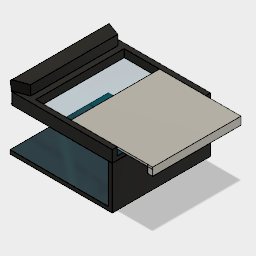
Hologram unit (Autodesk Fusion 360 design; units mm, degrees)
Autodesk Fusion 360 part; units mm, degrees
note: some values were not read from the file. Chosen so that the rebuilt part matches the saved one: that a step has no effect; the sign of a taper.
sketch "Sketch1" plane through (0, 0, 0) normal (0, 1, 0) x (1, 0, 0)
  line L0 (1.3, 0.4) -> (6.3, 0.4)
  line L1 (6.3, 0.4) -> (6.3, 5.4)
  line L2 (6.3, 5.4) -> (1.3, 5.4)
  line L3 (1.3, 5.4) -> (1.3, 0.4)
  dimension "d1" = 5
  dimension "d2" = 5
  measures "d1" distance of L0.start L0.end
  measures "d2" distance of L0.start L2.end
extrude "Extrude1" add sketch "Sketch1" along normal blind 2 draft -45 makes body 1
sketch "Sketch2" plane through (0, 0, 0) normal (0, -1, 0) x (1, 0, 0)
  line L0 (1.3, -0.4) -> (1.3, -5.4)
  line L1 (1.3, -5.4) -> (6.3, -5.4)
  line L2 (6.3, -5.4) -> (6.3, -0.4)
  line L3 (6.3, -0.4) -> (1.3, -0.4)
  line L4 (1.3, -0.4) -> (6.3, -0.4)
  line L5 (6.3, -0.4) -> (6.3, -5.4)
  line L6 (6.3, -5.4) -> (1.3, -5.4)
  line L7 (1.3, -5.4) -> (1.3, -0.4)
extrude "Extrude2" add sketch "Sketch2" along normal blind 0.2 bodies 1
extrude "Extrude3" add 1 faces at (6.3, -0.1333, -3.7333) along direction (1, 0, 0) blind 0.3 on bodies 1 bodies 1
extrude "Extrude4" add 1 faces at (6.4, 0, -2.0667) along direction (0, 1, 0) blind 2 on bodies 1 bodies 1
move_face "OffsetFaces1" offset -0.1 1 faces at (6.6, 1.2667, -3.7333) on bodies 1
sketch "Sketch1 (2)" plane through (0, -0.2, 0) normal (0, -1, 0) x (1, 0, 0) in component "Component"
  line L0 (1.3, -5.4) -> (6.5, -5.4)
  line L1 (6.5, -5.4) -> (6.5, -0.4)
  line L2 (6.5, -0.4) -> (1.3, -0.4)
  line L3 (1.3, -0.4) -> (1.3, -5.4)
  line L4 (1.3, -5.4) -> (6.5, -5.4)
  line L5 (6.5, -5.4) -> (6.5, -0.4)
  line L6 (6.5, -0.4) -> (1.3, -0.4)
  line L7 (1.3, -0.4) -> (1.3, -5.4)
extrude "Extrude1'" add sketch "Sketch1 (2)" along normal blind 0.3 separate body makes body 2 in component "Component"
move_face "OffsetFaces1'" offset 0.3 1 faces at (3.0333, -0.2, -2.0667) on bodies 2 in component "Component"
sketch "Sketch2 (2)" plane through (0, 0.1, 0) normal (0, 1, 0) x (-1, 0, 0) in component "Component"
  line L0 (-1.3, -5.4) -> (-1.3, -0.4)
  line L1 (-1.3, -0.4) -> (-6.5, -0.4)
  line L2 (-6.5, -0.4) -> (-6.5, -5.4)
  line L3 (-6.5, -5.4) -> (-1.3, -5.4)
  line L4 (-1.5531, -0.6531) -> (-6.2469, -0.6531)
  line L5 (-6.2469, -0.6531) -> (-6.2469, -5.1469)
  line L6 (-6.2469, -5.1469) -> (-1.5531, -5.1469)
  line L7 (-1.5531, -5.1469) -> (-1.5531, -0.6531)
  dimension "d17" = 0.2531
extrude "Extrude2'" cut sketch "Sketch2 (2)" against normal blind 0.4 contours L4 L5 L6 L7 bodies 2 in component "Component"
sketch "Sketch4" plane through (0, 2.2, 0) normal (0, 1, 0) x (-1, 0, 0)
  line L0 (-1.5531, -5.1469) -> (-1.5531, -0.6531)
  line L1 (-1.5531, -0.6531) -> (-6.2469, -0.6531)
  line L2 (-6.2469, -0.6531) -> (-6.2469, -5.1469)
  line L3 (-6.2469, -5.1469) -> (-1.5531, -5.1469)
  line L4 (-1.5531, -5.1469) -> (-2.3552, -5.1469)
  line L5 (-2.3552, -5.1469) -> (-2.3552, -0.6531)
  line L6 (-2.3552, -0.6531) -> (-1.5531, -0.6531)
  line L7 (-1.5531, -0.6531) -> (-1.5531, -5.1469)
extrude "Extrude3'" add sketch "Sketch4" along normal blind 0.4 contours L0 L1 L3 L4 L5 L6 L7 sketch seen with x (1, 0, 0) y (0, 1, 0) z (0, 0, 1) at (0, -2.5, 0) bodies 2 in component "Component"
sketch "Sketch5" plane through (0, 2.6, 0) normal (0, 1, 0) x (-1, 0, 0)
  line L0 (-6.2469, -0.6531) -> (-2.3552, -0.6531)
  line L1 (-2.3552, -0.6531) -> (-2.3552, -5.1469)
  line L2 (-2.3552, -5.1469) -> (-6.2469, -5.1469)
  line L3 (-6.2469, -5.1469) -> (-6.2469, -0.6531)
  line L4 (-1.3, -5.4) -> (-1.3, -0.4)
  line L5 (-1.3, -0.4) -> (-6.5, -0.4)
  line L6 (-6.5, -0.4) -> (-6.5, -5.4)
  line L7 (-6.5, -5.4) -> (-1.3, -5.4)
  line L8 (-6.2469, -5.1469) -> (-6.5, -5.1469)
  line L9 (-6.5, -5.1469) -> (-6.5, -0.6503)
  line L10 (-6.5, -0.6503) -> (-6.2469, -0.6503)
  line L11 (-6.2469, -0.6503) -> (-6.2469, -5.1469)
extrude "Extrude4'" cut sketch "Sketch5" against normal blind 0.4 contours L3 L6 L8 L9 L10 L11 sketch seen with x (1, 0, 0) y (0, 1, 0) z (0, 0, 1) at (0, -2.5, 0) bodies 2 in component "Component"
sketch "Sketch1 (3)" plane through (0, 2.6, 0) normal (0, 1, 0) x (-1, 0, 0) in component "Cover"
  line L0 (-6.5, -0.6503) -> (-6.2469, -0.6503)
  line L1 (-6.2469, -0.6503) -> (-6.2469, -0.6531)
  line L2 (-6.2469, -0.6531) -> (-2.3552, -0.6531)
  line L3 (-2.3552, -0.6531) -> (-2.3552, -5.1469)
  line L4 (-2.3552, -5.1469) -> (-6.5, -5.1469)
  line L5 (-6.5, -5.1469) -> (-6.5, -5.4)
  line L6 (-6.5, -5.4) -> (-1.3, -5.4)
  line L7 (-1.3, -5.4) -> (-1.3, -0.4)
  line L8 (-1.3, -0.4) -> (-6.5, -0.4)
  line L9 (-6.5, -0.4) -> (-6.5, -0.6503)
  line L10 (-2.3552, -5.1469) -> (-6.5, -5.1469)
  line L11 (-6.5, -5.1469) -> (-6.5, -0.6503)
  line L12 (-6.5, -0.6503) -> (-2.3552, -0.6503)
  line L13 (-2.3552, -0.6503) -> (-2.3552, -5.1469)
extrude "Extrude1''" add sketch "Sketch1 (3)" against normal blind 0.1 separate body contours L0 L1 L2 L3 L4 L10 L11 L12 L13 makes body 3 in component "Cover"
sketch "Sketch2 (3)" plane through (0, 2.5, 0) normal (0, -1, 0) x (1, 0, 0) in component "Cover"
  line L0 (6.2469, -0.6503) -> (6.2469, -0.6531)
  line L1 (6.2469, -0.6531) -> (2.3552, -0.6531)
  line L2 (2.3552, -0.6531) -> (2.3552, -5.1469)
  line L3 (2.3552, -5.1469) -> (6.5, -5.1469)
  line L4 (6.5, -5.1469) -> (6.5, -0.6503)
  line L5 (6.5, -0.6503) -> (6.2469, -0.6503)
  line L6 (6.2469, -0.6531) -> (6.5, -0.6531)
  line L7 (6.5, -0.6531) -> (6.5, -5.1469)
  line L8 (6.5, -5.1469) -> (6.2469, -5.1469)
  line L9 (6.2469, -5.1469) -> (6.2469, -0.6531)
extrude "Extrude2''" add sketch "Sketch2 (3)" along normal blind 0.3 contours L3 L4 L6 L7 L8 L9 bodies 3 in component "Cover"
move_body "Move1" bodies 3 to x (1, 0, 0) y (0, 1, 0) z (0, 0, 1) at (1.8, 0, 0) in component "Cover"
sketch "Sketch1 (4)" plane through (0, 2.6, 0) normal (0, 1, 0) x (-1, 0, 0) in component "Kinect"
  line L0 (-6.5, -0.6503) -> (-6.2469, -0.6503)
  line L1 (-6.2469, -0.6503) -> (-6.2469, -0.6531)
  line L2 (-6.2469, -0.6531) -> (-2.3552, -0.6531)
  line L3 (-2.3552, -0.6531) -> (-2.3552, -5.1469)
  line L4 (-2.3552, -5.1469) -> (-6.5, -5.1469)
  line L5 (-6.5, -5.1469) -> (-6.5, -5.4)
  line L6 (-6.5, -5.4) -> (-1.3, -5.4)
  line L7 (-1.3, -5.4) -> (-1.3, -0.4)
  line L8 (-1.3, -0.4) -> (-6.5, -0.4)
  line L9 (-6.5, -0.4) -> (-6.5, -0.6503)
  line L10 (-1.3, -5.4) -> (-2.069, -5.4)
  line L11 (-2.069, -5.4) -> (-2.069, -0.4)
  line L12 (-2.069, -0.4) -> (-1.3, -0.4)
  line L13 (-1.3, -0.4) -> (-1.3, -5.4)
extrude "Extrude1'''" add sketch "Sketch1 (4)" along normal blind 0.5 separate body contours L6 L7 L8 L10 L11 L12 L13 makes body 4 in component "Kinect"
form "Form1" [no effect] in component "Kinect"
draft "Draft2" angle -20 neutral plane through (1.3, 2.6, -5.4) pull (-1, 0, 0) 1 faces at (1.5563, 2.7667, -0.4) on bodies 4 in component "Kinect"
draft "Draft3" angle -20 neutral plane through (1.3, 2.6, -5.4) pull (-1, 0, 0) 1 faces at (1.8126, 2.7667, -5.4) on bodies 4 in component "Kinect"
draft "Draft4" angle 5 neutral plane through (0, 3.1, 0) pull (0, -1, 0) 1 faces at (1.3, 2.7667, -3.7333) on bodies 4 in component "Kinect"
fillet "Fillet1" radius 0.06 2 edges at (1.3, 3.1, -2.9) (1.3437, 2.6, -2.9) on bodies 4 in component "Kinect"
sketch "Sketch4 (2)" plane through (1.5593, 0.1364, 0) normal (-0.996195, -0.087156, 0) x (0, 0, 1) in component "Kinect"
  line L0 (-5.3858, 2.528) -> (-0.4142, 2.528)
  line L1 (-0.4142, 2.528) -> (-0.4021, 2.9094)
  line L2 (-0.4021, 2.9094) -> (-5.3979, 2.9094)
  line L3 (-5.3979, 2.9094) -> (-5.3858, 2.528)
  circle A0 centre (-4, 2.75) radius 0.15
  circle A1 centre (-2.85, 2.75) radius 0.15
  circle A2 centre (-2.3743, 2.7507) radius 0.15
  dimension "d41" = 0.3
  dimension "d42" = 0.3
  dimension "d43" = 0.3
  measures "d41" diameter of A0
  measures "d42" diameter of A1
  measures "d43" diameter of A2
extrude "Extrude3''" cut sketch "Sketch4 (2)" against normal blind 0.1 draft -30 contours A0 | A1 | A2 bodies 4 in component "Kinect"
fillet "Fillet1'" radius 0.1 1 edges at (1.3, -0.2, -0.4) on bodies 2 in component "Component"
fillet "Fillet2" radius 0.1 1 edges at (1.3, -0.2, -5.4) on bodies 2 in component "Component"
sketch "Sketch6" plane through (1.5593, 0.1364, 0) normal (-0.996195, -0.087156, 0) x (0, 0, 1)
  circle A0 centre (-4, 2.75) radius 0.15
  circle A1 centre (-2.85, 2.75) radius 0.15
  circle A2 centre (-2.3743, 2.7507) radius 0.15
  line L0 (-5.3858, 2.528) -> (-0.4142, 2.528)
  line L1 (-0.4142, 2.528) -> (-0.4021, 2.9094)
  line L2 (-0.4021, 2.9094) -> (-5.3979, 2.9094)
  line L3 (-5.3979, 2.9094) -> (-5.3858, 2.528)
  circle A3 centre (-4, 2.75) radius 0.15
  circle A4 centre (-4, 2.75) radius 0.15
  circle A5 centre (-2.85, 2.75) radius 0.15
  circle A6 centre (-2.3743, 2.7507) radius 0.15
  circle A7 centre (-3.55, 2.75) radius 0.0258
extrude "Extrude4''" cut sketch "Sketch6" against normal blind 0.01 contours A7 bodies 4 in component "Kinect"
sketch "Sketch1 (5)" plane through (0, 0, 0) normal (0, 1, 0) x (1, 0, 0) in component "Base"
  line L0 (6.5, 5.4) -> (1.3, 5.4)
  line L1 (1.3, 5.4) -> (1.3, 0.4)
  line L2 (1.3, 0.4) -> (6.5, 0.4)
  line L3 (6.5, 0.4) -> (6.5, 5.4)
  line L4 (6.5, 5.4) -> (6.3, 5.4)
  line L5 (6.3, 5.4) -> (6.3, 0.4)
  line L6 (6.3, 0.4) -> (6.5, 0.4)
  line L7 (6.5, 0.4) -> (6.5, 5.4)
  point P0 (6.5, 5.4)
  point P1 (1.3, 0.4)
  point P2 (6.3, 0.4)
extrude "Extrude1''''" add sketch "Sketch1 (5)" against normal blind 0.2 separate body contours L0 L1 L2 L5 makes body 5 in component "Base"
extrude "Extrude2'''" add 1 faces at (6.3, -0.0667, -3.7333) along direction (1, 0, 0) blind 0.2 on bodies 5 bodies 5 in component "Base"
sketch "Sketch2 (4)" plane through (0, 0, 0) normal (0, 1, 0) x (-1, 0, 0) in component "Base"
  line L0 (-1.3, -5.4) -> (-1.3, -0.4)
  line L1 (-1.3, -0.4) -> (-6.5, -0.4)
  line L2 (-6.5, -0.4) -> (-6.5, -5.4)
  line L3 (-6.5, -5.4) -> (-1.3, -5.4)
  line L4 (-6.5, -0.4) -> (-6.3, -0.4)
  line L5 (-6.3, -0.4) -> (-6.3, -5.4)
  line L6 (-6.3, -5.4) -> (-6.5, -5.4)
  line L7 (-6.5, -5.4) -> (-6.5, -0.4)
  point P0 (-6.3, -5.4)
extrude "Extrude3'''" add sketch "Sketch2 (4)" along normal blind 2 contours L1 L2 L3 L4 L5 L6 L7 bodies 5 in component "Base"
extrude "Extrude5" cut 1 faces at (6.3, 0.6667, -2.0667) along direction (1, 0, 0) blind 0.3 on bodies 1 bodies 1
extrude "Extrude6" cut 1 faces at (4.7667, -0.2, -2.0667) along direction (0, 1, 0) blind 0.2 on bodies 1 bodies 1
sketch "Sketch7" plane through (1.5593, 0.1364, 0) normal (-0.996195, -0.087156, 0) x (0, 0, 1)
  circle A0 centre (-3.55, 2.75) radius 0.0258
  circle A1 centre (-4, 2.75) radius 0.15
  circle A2 centre (-2.85, 2.75) radius 0.15
  circle A3 centre (-2.3743, 2.7507) radius 0.15
  line L0 (-5.3858, 2.528) -> (-0.4142, 2.528)
  line L1 (-0.4142, 2.528) -> (-0.4021, 2.9094)
  line L2 (-0.4021, 2.9094) -> (-5.3979, 2.9094)
  line L3 (-5.3979, 2.9094) -> (-5.3858, 2.528)
  circle A4 centre (-4, 2.75) radius 0.15
  circle A5 centre (-2.85, 2.75) radius 0.15
  circle A6 centre (-2.3743, 2.7507) radius 0.15
extrude "Extrude7" add sketch "Sketch7" along normal blind 0.01 separate body contours A1 A4 makes body 6
sketch "Sketch8" plane through (1.5593, 0.1364, 0) normal (-0.996195, -0.087156, 0) x (0, 0, 1)
  circle A0 centre (-3.55, 2.75) radius 0.0258
  circle A1 centre (-4, 2.75) radius 0.15
  circle A2 centre (-2.85, 2.75) radius 0.15
  circle A3 centre (-2.3743, 2.7507) radius 0.15
  line L0 (-5.3858, 2.528) -> (-0.4142, 2.528)
  line L1 (-0.4142, 2.528) -> (-0.4021, 2.9094)
  line L2 (-0.4021, 2.9094) -> (-5.3979, 2.9094)
  line L3 (-5.3979, 2.9094) -> (-5.3858, 2.528)
  circle A4 centre (-2.85, 2.75) radius 0.15
extrude "Extrude8" add sketch "Sketch8" along normal blind 0.01 separate body contours A2 A4 makes body 7
sketch "Sketch9" plane through (1.5593, 0.1364, 0) normal (-0.996195, -0.087156, 0) x (0, 0, 1)
  circle A0 centre (-3.55, 2.75) radius 0.0258
  circle A1 centre (-4, 2.75) radius 0.15
  circle A2 centre (-2.85, 2.75) radius 0.15
  circle A3 centre (-2.3743, 2.7507) radius 0.15
  line L0 (-5.3858, 2.528) -> (-0.4142, 2.528)
  line L1 (-0.4142, 2.528) -> (-0.4021, 2.9094)
  line L2 (-0.4021, 2.9094) -> (-5.3979, 2.9094)
  line L3 (-5.3979, 2.9094) -> (-5.3858, 2.528)
  circle A4 centre (-2.3743, 2.7507) radius 0.15
extrude "Extrude9" add sketch "Sketch9" along normal blind 0.01 separate body contours A3 A4 makes body 8
component "Component" placed x (1, 0, 0) y (0, 1, 0) z (0, 0, 1) at (0, 2.5, 0)
component "Cover" placed x (1, 0, 0) y (0, 1, 0) z (0, 0, 1) at (0, 0, 0)
component "Kinect" placed x (1, 0, 0) y (0, 1, 0) z (0, 0, 1) at (0, 0, 0)
component "Base" placed x (1, 0, 0) y (0, 1, 0) z (0, 0, 1) at (0, 0, 0)
